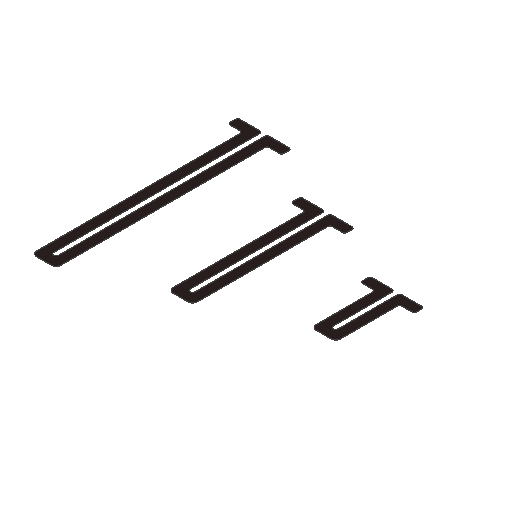
# Autodesk Inventor part: SensoriColorati
Saved by Autodesk Inventor 2025.4 (Build 294407000, 407)
## iProperties
Created: 2026-04-21
Part Number: SensoriColorati
Material: Generic
Document SubType Name: Modeling
Designer: gdira
Density: 1 g/cm^3
Appearance: Default
Author: gdira
Autodesk Inventor part; units mm, degrees
ref_plane "YZ Plane" through (0, 0, 0) normal (1, 0, 0) x (0, 1, 0)
ref_plane "XZ Plane" through (0, 0, 0) normal (0, 1, 0) x (-1, 0, 0)
ref_plane "XY Plane" through (0, 0, 0) normal (0, 0, 1) x (1, 0, 0)
sketch "Sketch1" plane through (0, 0, 0) normal (0, 1, 0) x (-1, 0, 0)
  arc A0 (-5.3961, 42.9951) -> (-7.3961, 40.9951) centre (-5.3961, 40.9951) ccw
  arc A1 (2.6039, 40.9951) -> (0.6039, 42.9951) centre (0.6039, 40.9951) ccw
  line L0 (-5.3961, 42.9951) -> (0.6039, 42.9951)
  line L1 (-2.3961, 38.9951) -> (-2.3961, 38.9951)
  arc A2 (-2.3961, 38.9951) -> (-3.3961, 37.9951) centre (-2.3961, 37.9951) ccw
  arc A3 (-1.3961, 37.9951) -> (-2.3961, 38.9951) centre (-2.3961, 37.9951) ccw
  line L2 (2.6039, 40.9951) -> (2.6039, -38.9794)
  line L3 (-7.3961, 40.9951) -> (-7.3961, -39.0072)
  line L4 (2.6039, -41.9976) -> (2.6039, -35.4252)
  line L5 (-7.3961, -42.0072) -> (-7.3961, -39.0072)
  arc A4 (-8.3961, -43.0072) -> (-7.3961, -42.0072) centre (-8.3961, -42.0072) ccw
  line L6 (-3.3961, 37.9951) -> (-3.3961, -46.0072)
  line L7 (-1.3961, -46.0104) -> (-1.3961, 37.9951)
  line L8 (-4.3961, -47.0072) -> (-12.3961, -47.0072)
  line L9 (-12.3961, -43.0072) -> (-8.3961, -43.0072)
  arc A5 (-12.3961, -43.0072) -> (-13.3961, -44.0072) centre (-12.3961, -44.0072) ccw
  line L10 (-13.3961, -46.0072) -> (-13.3961, -44.0072)
  arc A6 (-13.3961, -46.0072) -> (-12.3961, -47.0072) centre (-12.3961, -46.0072) ccw
  arc A7 (-1.3961, -46.0104) -> (-0.3961, -47.0104) centre (-0.3961, -46.0104) ccw
  arc A8 (-4.3961, -47.0072) -> (-3.3961, -46.0072) centre (-4.3961, -46.0072) ccw
  line L11 (1.5945, -47.0104) -> (-0.3961, -47.0104)
  line L12 (1.5945, -47.0104) -> (7.6057, -46.9994)
  line L13 (8.6039, -45.9994) -> (8.6039, -43.9976)
  line L14 (7.6039, -42.9976) -> (3.6039, -42.9976)
  arc A9 (7.6057, -46.9994) -> (8.6039, -45.9994) centre (7.6039, -45.9994) ccw
  arc A10 (8.6039, -43.9976) -> (7.6039, -42.9976) centre (7.6039, -43.9976) ccw
  arc A11 (2.6039, -41.9976) -> (3.6039, -42.9976) centre (3.6039, -41.9976) ccw
  arc A12 (-42.1557, -30.9546) -> (-41.1557, -31.9546) centre (-41.1557, -30.9546) ccw
  line L15 (-39.165, -31.9546) -> (-41.1557, -31.9546)
  line L16 (-38.1557, -26.9419) -> (-38.1557, -20.3695)
  arc A13 (-38.1557, -26.9419) -> (-37.1557, -27.9419) centre (-37.1557, -26.9419) ccw
  line L17 (-39.165, -31.9546) -> (-33.1539, -31.9437)
  line L18 (-33.1557, -27.9419) -> (-37.1557, -27.9419)
  arc A14 (-32.1557, -28.9419) -> (-33.1557, -27.9419) centre (-33.1557, -28.9419) ccw
  line L19 (-32.1557, -30.9437) -> (-32.1557, -28.9419)
  arc A15 (-33.1539, -31.9437) -> (-32.1557, -30.9437) centre (-33.1557, -30.9437) ccw
  arc A16 (-45.1557, -31.9515) -> (-44.1557, -30.9515) centre (-45.1557, -30.9515) ccw
  line L20 (-45.1557, -31.9515) -> (-53.1557, -31.9515)
  line L21 (-54.1557, -30.9515) -> (-54.1557, -28.9515)
  line L22 (-53.1557, -27.9515) -> (-49.1557, -27.9515)
  line L23 (-48.1557, -26.9515) -> (-48.1557, -23.9515)
  arc A17 (-49.1557, -27.9515) -> (-48.1557, -26.9515) centre (-49.1557, -26.9515) ccw
  arc A18 (-54.1557, -30.9515) -> (-53.1557, -31.9515) centre (-53.1557, -30.9515) ccw
  arc A19 (-53.1557, -27.9515) -> (-54.1557, -28.9515) centre (-53.1557, -28.9515) ccw
  line L24 (-44.1557, 23.0508) -> (-44.1557, -30.9515)
  line L25 (-42.1557, -30.9546) -> (-42.1557, 23.0508)
  line L26 (-43.1557, 24.0508) -> (-43.1557, 24.0508)
  line L27 (-48.1557, 26.0508) -> (-48.1557, -23.9515)
  line L28 (-46.1557, 28.0508) -> (-40.1557, 28.0508)
  line L29 (-38.1557, 26.0508) -> (-38.1557, -23.9237)
  arc A20 (-46.1557, 28.0508) -> (-48.1557, 26.0508) centre (-46.1557, 26.0508) ccw
  arc A21 (-38.1557, 26.0508) -> (-40.1557, 28.0508) centre (-40.1557, 26.0508) ccw
  arc A22 (-42.1557, 23.0508) -> (-43.1557, 24.0508) centre (-43.1557, 23.0508) ccw
  arc A23 (-43.1557, 24.0508) -> (-44.1557, 23.0508) centre (-43.1557, 23.0508) ccw
  line L30 (-81.4368, -18.0467) -> (-83.4318, -18.0382)
  line L31 (-87.4275, -18.0436) -> (-95.4275, -18.0436)
  line L32 (-81.4368, -18.0467) -> (-75.4257, -18.0358)
  line L33 (-86.4275, 6.9587) -> (-86.4275, -17.0436)
  line L34 (-84.4275, -17.0382) -> (-84.4275, 6.9587)
  line L35 (-85.4275, 7.9587) -> (-85.4275, 7.9587)
  line L36 (-90.4275, 9.9587) -> (-90.4275, -10.0436)
  line L37 (-88.4275, 11.9587) -> (-82.4275, 11.9587)
  line L38 (-80.4275, 9.9587) -> (-80.4275, -10.0158)
  arc A24 (-88.4275, 11.9587) -> (-90.4275, 9.9587) centre (-88.4275, 9.9587) ccw
  arc A25 (-80.4275, 9.9587) -> (-82.4275, 11.9587) centre (-82.4275, 9.9587) ccw
  line L39 (-74.4275, -17.0358) -> (-74.4275, -15.034)
  line L40 (-75.4275, -14.034) -> (-79.4275, -14.034)
  line L41 (-80.4275, -13.034) -> (-80.4275, -6.4616)
  line L42 (-96.4275, -17.0436) -> (-96.4275, -15.0436)
  line L43 (-95.4275, -14.0436) -> (-91.4275, -14.0436)
  line L44 (-90.4275, -13.0436) -> (-90.4275, -10.0436)
  arc A26 (-91.4275, -14.0436) -> (-90.4275, -13.0436) centre (-91.4275, -13.0436) ccw
  arc A27 (-95.4275, -14.0436) -> (-96.4275, -15.0436) centre (-95.4275, -15.0436) ccw
  arc A28 (-96.4275, -17.0436) -> (-95.4275, -18.0436) centre (-95.4275, -17.0436) ccw
  arc A29 (-87.4275, -18.0436) -> (-86.4275, -17.0436) centre (-87.4275, -17.0436) ccw
  arc A30 (-84.4275, -17.0382) -> (-83.4318, -18.0382) centre (-83.4275, -17.0382) ccw
  arc A31 (-75.4257, -18.0358) -> (-74.4275, -17.0358) centre (-75.4275, -17.0358) ccw
  arc A32 (-74.4275, -15.034) -> (-75.4275, -14.034) centre (-75.4275, -15.034) ccw
  arc A33 (-80.4275, -13.034) -> (-79.4275, -14.034) centre (-79.4275, -13.034) ccw
  arc A34 (-85.4275, 7.9587) -> (-86.4275, 6.9587) centre (-85.4275, 6.9587) ccw
  arc A35 (-84.4275, 6.9587) -> (-85.4275, 7.9587) centre (-85.4275, 6.9587) ccw
  point P0 (0, 0)
  point P1 (1.3964, -43.0157)
  point P2 (-2.3961, 38.9951)
  point P3 (2.2842, -26.5744)
  point P4 (-1.3961, -47.0104)
  point P5 (-13.3961, -47.0072)
  point P6 (-13.3961, -43.0072)
  point P7 (4.6001, -47.0049)
  point P8 (8.6039, -46.9976)
  point P9 (8.6039, -42.9976)
  point P10 (-40.3838, -15.9392)
  point P11 (-42.1557, -31.9546)
  point P12 (-36.1594, -31.9492)
  point P13 (-32.1557, -31.9419)
  point P14 (-32.1557, -27.9419)
  point P15 (-54.1557, -31.9515)
  point P16 (-54.1557, -27.9515)
  point P17 (-38.4753, -11.5187)
  point P18 (-43.1557, 24.0508)
  point P19 (-43.1557, 28.0508)
  point P20 (-80.7471, 2.3892)
  point P21 (-84.4275, -18.034)
  point P22 (-78.4312, -18.0413)
  point P23 (-96.4275, -18.0436)
  point P24 (-74.4275, -18.034)
  point P25 (-85.4275, 11.9587)
  point P26 (-74.4275, -14.034)
  point P27 (-96.4275, -14.0436)
  point P28 (-80.4275, -10.0158)
  point P29 (-85.4275, 7.9587)
  point P30 (-43.1557, 24.0508)
  dimension "d0" = 10
  dimension "d1" = 4
  dimension "d2" = 4
  dimension "d3" = 2
  dimension "d5" = 90
  dimension "d6" = 2
  dimension "d7" = 4
  dimension "d8" = 4
  dimension "d9" = 1
  dimension "d10" = 1
  dimension "d11" = 10
  dimension "d12" = 4
  dimension "d13" = 4
  dimension "d14" = 2
  dimension "d15" = 4
  dimension "d16" = 60
  dimension "d17" = 2
  dimension "d18" = 4
  dimension "d19" = 4
  dimension "d20" = 1
  dimension "d21" = 1
  dimension "d22" = 10
  dimension "d23" = 4
  dimension "d24" = 4
  dimension "d25" = 2
  dimension "d26" = 4
  dimension "d27" = 30
  dimension "d28" = 2
  dimension "d29" = 4
  dimension "d30" = 4
  dimension "d31" = 1
  dimension "d32" = 1
  constraints: 90 end point, 72 point on circle, 72 tangent, 36 centre point, 33 point on line, 27 equal radius, 15 perpendicular, 8 midpoint, 6 horizontal, 6 vertical, 3 collinear, 3 parallel
  measures "d0" distance of point (8.604, -46.998) point (-1.396, -47.01)
  measures "d1" distance between parallel lines of L7 L2
  measures "d2" distance between parallel lines of L3 L6
  measures "d3" distance between parallel lines of L6 L7
  measures "d5" distance from line of point (4.6, -47.005) L0
  measures "d6" radius of A0
  measures "d7" distance of point (8.604, -46.998) point (8.604, -42.998)
  measures "d8" distance of point (-13.396, -47.007) point (-13.396, -43.007)
  measures "d9" radius of A4
  measures "d10" radius of A2
  measures "d11" distance of point (-32.156, -31.942) point (-42.156, -31.955)
  measures "d12" distance between parallel lines of L25 L29
  measures "d13" distance between parallel lines of L27 L24
  measures "d14" distance between parallel lines of L24 L25
  measures "d15" distance of point (-43.156, 28.051) point (-43.156, 24.051)
  measures "d16" distance from line of point (-36.159, -31.949) L28
  measures "d17" radius of A20
  measures "d18" distance of point (-32.156, -31.942) point (-32.156, -27.942)
  measures "d19" distance of point (-54.156, -31.951) point (-54.156, -27.951)
  measures "d20" radius of A17
  measures "d21" radius of A23
  measures "d22" distance of point (-74.428, -18.034) point (-84.428, -18.034)
  measures "d23" distance between parallel lines of L34 L38
  measures "d24" distance between parallel lines of L36 L33
  measures "d25" distance between parallel lines of L33 L34
  measures "d26" distance of point (-85.428, 11.959) point (-85.428, 7.959)
  measures "d27" distance from line of point (-78.431, -18.041) L37
  measures "d28" radius of A24
  measures "d29" distance of point (-74.428, -18.034) point (-74.428, -14.034)
  measures "d30" distance of point (-96.428, -18.044) point (-96.428, -14.044)
  measures "d31" radius of A26
  measures "d32" radius of A34
extrude "Extrusion1" add sketch "Sketch1" along normal blind 0.15
body "Solid1"
